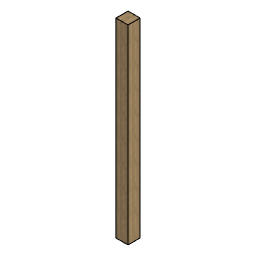
esqueleto totem v5 (Autodesk Fusion 360 archive; units mm, degrees)
design "Liston 30cm"
Autodesk Fusion 360 part; units mm, degrees
sketch "Boceto1" plane through (0, 0, 0) normal (0, 0, 1) x (1, 0, 0)
  line L0 (0, 0) -> (19, 0)
  line L1 (19, 0) -> (19, 19)
  line L2 (19, 19) -> (0, 19)
  line L3 (0, 19) -> (0, 0)
  dimension "d1" = 19
  dimension "d2" = 19
  constraint horizontal L0
  constraint vertical L1
  constraint horizontal L2
  constraint vertical L3
  constraint coincident L0.start L3.end
  measures "d1" distance of L0.start L0.end
  measures "d2" distance of L0.start L2.end
extrude "Extruir1" add sketch "Boceto1" along normal blind 300

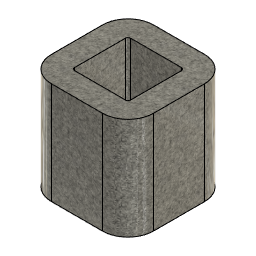
design "Adocreto"
Autodesk Fusion 360 part; units mm, degrees
sketch "Boceto1" plane through (0, 0, 0) normal (0, 0, 1) x (1, 0, 0)
  line L0 (50, 0) -> (150, 0)
  line L1 (200, 50) -> (200, 150)
  line L2 (150, 200) -> (50, 200)
  line L3 (0, 150) -> (0, 50)
  arc A0 (50, 200) -> (0, 150) centre (50, 150) ccw
  arc A1 (200, 150) -> (150, 200) centre (150, 150) ccw
  arc A2 (150, 0) -> (200, 50) centre (150, 50) ccw
  arc A3 (0, 50) -> (50, 0) centre (50, 50) ccw
  line L4 (45, 150) -> (45, 50)
  arc A4 (45, 50) -> (50, 45) centre (50, 50) ccw
  line L5 (50, 45) -> (150, 45)
  arc A5 (150, 45) -> (155, 50) centre (150, 50) ccw
  line L6 (155, 50) -> (155, 150)
  arc A6 (155, 150) -> (150, 155) centre (150, 150) ccw
  line L7 (150, 155) -> (50, 155)
  arc A7 (50, 155) -> (45, 150) centre (50, 150) ccw
  point P0 (200, 0)
  point P1 (0, 200)
  dimension "d1" = 200
  dimension "d2" = 200
  dimension "d3" = 50
  dimension "d4" = -45
  constraint horizontal L0
  constraint vertical L1
  constraint horizontal L2
  constraint vertical L3
  constraint coincident P1 L2
  constraint coincident P1 L3
  constraint tangent L2 A0
  constraint tangent L3 A0
  constraint tangent L2 A1
  constraint tangent L1 A1
  constraint equal A0 A1
  constraint coincident P0 L1
  constraint coincident P0 L0
  constraint tangent L1 A2
  constraint tangent L0 A2
  constraint equal A0 A2
  constraint coincident origin L0
  constraint coincident origin L3
  constraint tangent L0 A3
  constraint tangent L3 A3
  constraint equal A0 A3
  measures "d1" distance of origin P0
  measures "d2" distance of origin P1
  measures "d3" radius of A0
extrude "Extruir1" add sketch "Boceto1" along normal blind 200

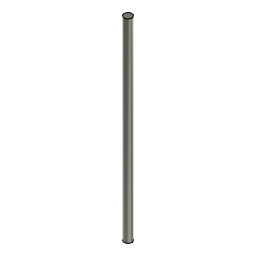
design "eje"
Autodesk Fusion 360 part; units mm, degrees
sketch "Boceto1" plane through (0, 0, 0) normal (0, 0, 1) x (1, 0, 0)
  circle A0 centre (0, 0) radius 6
  dimension "d1" = 12
  constraint coincident A0.centre origin
  measures "d1" diameter of A0
extrude "Extruir1" add sketch "Boceto1" along normal blind 300

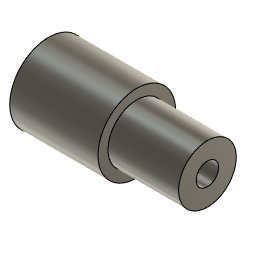
design "pieza motor s v1"
Autodesk Fusion 360 part; units mm, degrees
sketch "Boceto1" plane through (0, 0, 0) normal (1, 0, 0) x (0, 1, 0)
  circle A0 centre (4.4228, -4.6349) radius 3.175
  circle A1 centre (4.4228, -4.6349) radius 8.175
  dimension "d1" = 6.35
  dimension "d2" = 5
  measures "d1" diameter of A0
extrude "Extruir1" add sketch "Boceto1" along normal blind 15
sketch "Boceto2" plane through (0, 0, 0) normal (-1, 0, 0) x (0, -1, 0)
  circle A0 centre (-4.4228, -4.6349) radius 3.175
  circle A1 centre (-4.4228, -4.6349) radius 8.175
  circle A2 centre (-4.4228, -4.6349) radius 8.175
  constraint concentric A0 A2
extrude "Extruir2" add sketch "Boceto2" along normal blind 5 contours A0 | A1 A2
sketch "Boceto3" plane through (-5, 0, 0) normal (-1, 0, 0) x (0, -1, 0)
  circle A0 centre (-4.4228, -4.6349) radius 8.175
  circle A1 centre (-4.4228, -4.6349) radius 11
  dimension "d7" = 22
  constraint concentric A0 A1
  measures "d7" diameter of A1
extrude "Extruir3" add sketch "Boceto3" along normal blind 25 contours A0 | A1
sketch "Boceto4" plane through (-30, 0, 0) normal (-1, 0, 0) x (0, -1, 0)
  circle A0 centre (-4.4228, -4.6349) radius 11
  circle A1 centre (-4.4228, -4.6349) radius 6
  dimension "d10" = 12
  constraint concentric A0 A1
  measures "d10" diameter of A1
extrude "Extruir4" cut sketch "Boceto4" against normal blind 23 contours A1

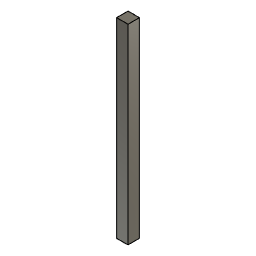
design "Liston marco"
Autodesk Fusion 360 part; units mm, degrees
sketch "Boceto1" plane through (0, 0, 0) normal (0, 0, 1) x (1, 0, 0)
  line L0 (0, 0) -> (19, 0)
  line L1 (19, 0) -> (19, 19)
  line L2 (19, 19) -> (0, 19)
  line L3 (0, 19) -> (0, 0)
  dimension "d1" = 19
  dimension "d2" = 19
  constraint horizontal L0
  constraint vertical L1
  constraint horizontal L2
  constraint vertical L3
  constraint coincident L0.start L3.end
  measures "d1" distance of L0.start L0.end
  measures "d2" distance of L0.start L2.end
extrude "Extruir1" add sketch "Boceto1" along normal blind 319

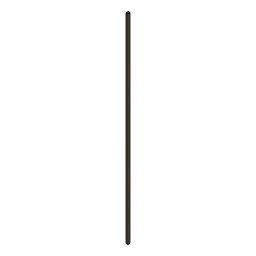
design "Liston 2m"
Autodesk Fusion 360 part; units mm, degrees
sketch "Boceto1" plane through (0, 0, 0) normal (0, 0, 1) x (1, 0, 0)
  line L0 (0, 0) -> (19, 0)
  line L1 (19, 0) -> (19, 19)
  line L2 (19, 19) -> (0, 19)
  line L3 (0, 19) -> (0, 0)
  dimension "d1" = 19
  dimension "d2" = 19
  constraint horizontal L0
  constraint vertical L1
  constraint horizontal L2
  constraint vertical L3
  constraint coincident L0.start L3.end
  measures "d1" distance of L0.start L0.end
  measures "d2" distance of L0.start L2.end
extrude "Extruir1" add sketch "Boceto1" along normal blind 2000
